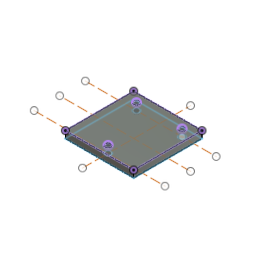
bearing_plate (Autodesk Fusion 360 design; units mm, degrees)
Autodesk Fusion 360 part; units mm, degrees
sketch "Sketch1" plane through (0, 0, 0) normal (0, 1, 0) x (1, 0, 0)
  line L0 (-50, 25) -> (10, 25)
  line L1 (10, 25) -> (10, -35)
  line L2 (10, -35) -> (-50, -35)
  line L3 (-50, -35) -> (-50, 25)
  line L4 (-20, -50) -> (-20, 45) construction
  line L5 (30, -5) -> (-85, -5) construction
  line L6 (-85, 17.5) -> (30, 17.5) construction
  line L7 (-85, -27.5) -> (30, -27.5) construction
  circle A0 centre (-40, 17.5) radius 2.55
  circle A1 centre (0, 17.5) radius 2.55
  circle A2 centre (-20, -27.5) radius 2.55
  dimension "d1" = 60
  dimension "d2" = 60
  dimension "d3" = 22.5
  dimension "d4" = 5.1
  dimension "d5" = 5.1
  constraint horizontal L0
  constraint vertical L1
  constraint horizontal L2
  constraint vertical L3
  constraint perpendicular L0 L4
  constraint perpendicular L1 L5
  constraint perpendicular L1 L6
  constraint symmetric L5 L6.start L7.start
  constraint symmetric L5 L6.end L7.end
  constraint coincident L6 A0.centre
  constraint symmetric L4 A0 A1
  constraint coincident L7 A2.centre
  constraint coincident L4 A2.centre
  measures "d1" distance of L0.start L2.end
  measures "d2" distance of L0.start L0.end
  measures "d3" distance of L5 L6
  measures "d4" diameter of A0
  measures "d5" diameter of A2
extrude "Extrude1" add sketch "Sketch1" along normal blind 6
sketch "Sketch3" plane through (0, 6, 0) normal (0, 1, 0) x (-1, 0, 0)
  circle A0 centre (40, -17.5) radius 2.55
  circle A1 centre (20, 27.5) radius 2.55
  circle A2 centre (0, -17.5) radius 2.55
  line L0 (50, 35) -> (-10, 35)
  line L1 (-10, 35) -> (-10, -25)
  line L2 (-10, -25) -> (50, -25)
  line L3 (50, -25) -> (50, 35)
equation "d3 = separation / 2"
equation "d4 = hole_01"
equation "d5 = hole_01"
equation "separation = 45 mm"
equation "hole_01 = 5.1 mm"
